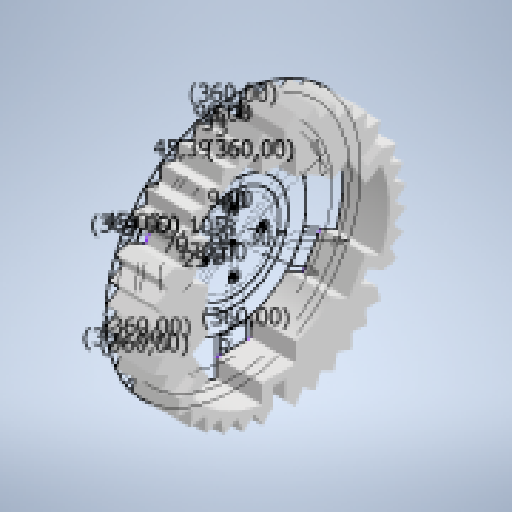
# Autodesk Inventor part: wheel
Saved by Autodesk Inventor 2023 (Build 270158000, 158)
## iProperties
Created: 2026-02-20
Part Number: wheel
Material: Типовые
Document SubType Name: Modeling
Designer: garin
Density: 1 g/cm^3
Appearance: По умолчанию
Author: garin
Autodesk Inventor part; units mm, degrees
ref_plane "YZ Plane" through (0, 0, 0) normal (1, 0, 0) x (0, 1, 0)
ref_plane "XZ Plane" through (0, 0, 0) normal (0, 1, 0) x (-1, 0, 0)
ref_plane "XY Plane" through (0, 0, 0) normal (0, 0, 1) x (1, 0, 0)
ref_plane "РабПлоскость1" through (-2, -29.6838, -23.3604) normal (-1, 0, 0) x (0, 0, 1)
sketch "Эскиз1" plane through (0, 0, 0) normal (1, 0, 0) x (0, 1, 0)
  circle A0 centre (0, 0) radius 35
  circle A1 centre (0, 0) radius 20
  line L0 (0, 0) -> (34.5691, 5.4752) construction
  line L1 (0, 0) -> (35, 0) construction
  line L2 (0, 0) -> (34.5691, -5.4752) construction
  line L3 (34.5691, 5.4752) -> (29.6307, 4.693) construction
  line L4 (29.6307, 4.693) -> (19.4416, 4.693)
  line L5 (19.4416, 4.693) -> (34.6839, 4.693)
  line L6 (19.4416, -4.693) -> (34.6839, -4.693)
  line L7 (13.7851, 14.4904) -> (21.4063, 27.6907) construction
  line L8 (10.751, 28.0074) -> (5.6565, 19.1834) construction
  line L9 (5.6565, 19.1834) -> (13.2777, 32.3837) construction
  line L10 (-5.6565, 19.1834) -> (-13.2777, 32.3837) construction
  line L11 (-18.8796, 23.3144) -> (-13.7851, 14.4904) construction
  line L12 (-13.7851, 14.4904) -> (-21.4063, 27.6907) construction
  line L13 (-19.4416, 4.693) -> (-34.6839, 4.693) construction
  line L14 (-29.6307, -4.693) -> (-19.4416, -4.693) construction
  line L15 (-19.4416, -4.693) -> (-34.6839, -4.693) construction
  line L16 (-13.7851, -14.4904) -> (-21.4063, -27.6907) construction
  line L17 (-10.751, -28.0074) -> (-5.6565, -19.1834) construction
  line L18 (-5.6565, -19.1834) -> (-13.2777, -32.3837) construction
  line L19 (5.6565, -19.1834) -> (13.2777, -32.3837) construction
  line L20 (18.8796, -23.3144) -> (13.7851, -14.4904) construction
  line L21 (13.7851, -14.4904) -> (21.4063, -27.6907) construction
  line L22 (0, 0) -> (17.5, 30.3109) construction
  line L23 (0, 0) -> (-17.5, 30.3109) construction
  line L24 (0, 0) -> (-35, 0) construction
  line L25 (0, 0) -> (-17.5, -30.3109) construction
  line L26 (0, 0) -> (17.5, -30.3109) construction
  line L27 (34.6839, 4.693) -> (29.6839, 4.693) construction
  line L28 (29.6839, 4.693) -> (29.6839, -4.693)
  line L29 (29.6839, 4.693) -> (29.6839, 1.693)
  line L30 (29.6839, 1.693) -> (34.959, 1.693)
  line L31 (29.6839, -4.693) -> (29.6839, -1.693) construction
  line L32 (29.6839, -1.693) -> (34.959, -1.693)
  line L33 (13.7851, 14.4904) -> (21.4063, 27.6907)
  line L34 (10.751, 28.0074) -> (5.6565, 19.1834)
  line L35 (13.3758, 26.5536) -> (16.0133, 31.1219)
  line L36 (5.6565, 19.1834) -> (13.2777, 32.3837)
  line L37 (10.7777, 28.0536) -> (18.9063, 23.3605)
  line L38 (16.3082, 24.8605) -> (18.9457, 29.4289)
  line L39 (-5.6565, 19.1834) -> (-13.2777, 32.3837)
  line L40 (-18.8796, 23.3144) -> (-13.7851, 14.4904)
  line L41 (-16.3082, 24.8605) -> (-18.9457, 29.4289)
  line L42 (-13.7851, 14.4904) -> (-21.4063, 27.6907)
  line L43 (-18.9063, 23.3605) -> (-10.7777, 28.0536)
  line L44 (-13.3758, 26.5536) -> (-16.0133, 31.1219)
  line L45 (-19.4416, 4.693) -> (-34.6839, 4.693)
  line L46 (-29.6307, -4.693) -> (-19.4416, -4.693)
  line L47 (-29.6839, -1.693) -> (-34.959, -1.693)
  line L48 (-19.4416, -4.693) -> (-34.6839, -4.693)
  line L49 (-29.6839, -4.693) -> (-29.6839, 4.693)
  line L50 (-29.6839, 1.693) -> (-34.959, 1.693)
  line L51 (-13.7851, -14.4904) -> (-21.4063, -27.6907)
  line L52 (-10.751, -28.0074) -> (-5.6565, -19.1834)
  line L53 (-13.3758, -26.5536) -> (-16.0133, -31.1219)
  line L54 (-5.6565, -19.1834) -> (-13.2777, -32.3837)
  line L55 (-10.7777, -28.0536) -> (-18.9063, -23.3605)
  line L56 (-16.3082, -24.8605) -> (-18.9457, -29.4289)
  line L57 (5.6565, -19.1834) -> (13.2777, -32.3837)
  line L58 (18.8796, -23.3144) -> (13.7851, -14.4904)
  line L59 (16.3082, -24.8605) -> (18.9457, -29.4289)
  line L60 (13.7851, -14.4904) -> (21.4063, -27.6907)
  line L61 (18.9063, -23.3605) -> (10.7777, -28.0536)
  line L62 (13.3758, -26.5536) -> (16.0133, -31.1219)
  circle A2 centre (0, 0) radius 30.0525
  line L63 (21.4063, 27.6907) -> (19.9063, 25.0926) construction
  line L64 (18.9457, 29.4289) -> (17.4457, 26.8308) construction
  line L65 (17.4457, 26.8308) -> (21.2118, 27.8399)
  line L66 (0, 0) -> (21.2118, 27.8399) construction
  line L67 (21.2384, 23.9411) -> (21.2118, 27.8399)
  line L68 (24.7499, 20.2901) -> (25.3388, 24.1443)
  line L69 (21.4607, 23.742) -> (25.3388, 24.1443)
  line L70 (27.6414, 16.1308) -> (28.831, 19.8437)
  line L71 (24.938, 20.0584) -> (28.831, 19.8437)
  line L72 (29.8403, 11.5673) -> (31.6009, 15.046)
  line L73 (27.7906, 15.8723) -> (31.6009, 15.046)
  line L74 (31.2917, 6.714) -> (33.5791, 9.8714)
  line L75 (29.9469, 11.2885) -> (33.5791, 9.8714)
  line L76 (31.9591, 1.6925) -> (34.716, 4.4494)
  line L77 (31.3529, 6.4219) -> (34.716, 4.4494)
  circle A3 centre (0, 0) radius 32.0038
  line L78 (-14.5133, 28.5238) -> (-13.5042, 32.2899)
  line L79 (-10.1144, 30.3635) -> (-13.5042, 32.2899)
  line L80 (-9.8308, 30.4565) -> (-8.2401, 34.0162)
  line L81 (-5.1968, 31.5791) -> (-8.2401, 34.0162)
  line L82 (14.5138, 28.5236) -> (13.5047, 32.2897)
  line L83 (10.1149, 30.3634) -> (13.5047, 32.2897)
  line L84 (9.8313, 30.4564) -> (8.2407, 34.016)
  line L85 (5.1973, 31.579) -> (8.2407, 34.016)
  line L86 (4.9026, 31.6261) -> (2.7702, 34.8902)
  line L87 (0.1495, 32.0035) -> (2.7702, 34.8902)
  line L88 (-0.149, 32.0035) -> (-2.7697, 34.8902)
  line L89 (-4.9021, 31.6262) -> (-2.7697, 34.8902)
  line L90 (-31.959, 1.693) -> (-34.716, 4.45)
  line L91 (-31.3528, 6.4224) -> (-34.716, 4.45)
  line L92 (-31.2916, 6.7145) -> (-33.5789, 9.8719)
  line L93 (-29.9467, 11.289) -> (-33.5789, 9.8719)
  line L94 (-17.4453, 26.8311) -> (-21.2113, 27.8403)
  line L95 (-21.238, 23.9415) -> (-21.2113, 27.8403)
  line L96 (-21.4603, 23.7424) -> (-25.3384, 24.1447)
  line L97 (-24.7496, 20.2905) -> (-25.3384, 24.1447)
  line L98 (-24.9377, 20.0588) -> (-28.8307, 19.8442)
  line L99 (-27.6411, 16.1312) -> (-28.8307, 19.8442)
  line L100 (-27.7903, 15.8727) -> (-31.6007, 15.0465)
  line L101 (-29.8401, 11.5678) -> (-31.6007, 15.0465)
  line L102 (-17.4457, -26.8308) -> (-21.2118, -27.8399)
  line L103 (-21.2384, -23.9411) -> (-21.2118, -27.8399)
  line L104 (-21.4607, -23.742) -> (-25.3388, -24.1443)
  line L105 (-24.7499, -20.2901) -> (-25.3388, -24.1443)
  line L106 (-31.9591, -1.6925) -> (-34.716, -4.4494)
  line L107 (-31.3529, -6.4219) -> (-34.716, -4.4494)
  line L108 (-31.2917, -6.714) -> (-33.5791, -9.8714)
  line L109 (-29.9469, -11.2885) -> (-33.5791, -9.8714)
  line L110 (-29.8403, -11.5673) -> (-31.6009, -15.046)
  line L111 (-27.7906, -15.8723) -> (-31.6009, -15.046)
  line L112 (-27.6414, -16.1308) -> (-28.831, -19.8437)
  line L113 (-24.938, -20.0584) -> (-28.831, -19.8437)
  line L114 (14.5133, -28.5238) -> (13.5042, -32.2899)
  line L115 (10.1144, -30.3635) -> (13.5042, -32.2899)
  line L116 (9.8308, -30.4565) -> (8.2401, -34.0162)
  line L117 (5.1968, -31.5791) -> (8.2401, -34.0162)
  line L118 (-14.5138, -28.5236) -> (-13.5047, -32.2897)
  line L119 (-10.1149, -30.3634) -> (-13.5047, -32.2897)
  line L120 (-9.8313, -30.4564) -> (-8.2407, -34.016)
  line L121 (-5.1973, -31.579) -> (-8.2407, -34.016)
  line L122 (-4.9026, -31.6261) -> (-2.7702, -34.8902)
  line L123 (-0.1495, -32.0035) -> (-2.7702, -34.8902)
  line L124 (0.149, -32.0035) -> (2.7697, -34.8902)
  line L125 (4.9021, -31.6262) -> (2.7697, -34.8902)
  line L126 (31.959, -1.693) -> (34.716, -4.45)
  line L127 (31.3528, -6.4224) -> (34.716, -4.45)
  line L128 (31.2916, -6.7145) -> (33.5789, -9.8719)
  line L129 (29.9467, -11.289) -> (33.5789, -9.8719)
  line L130 (17.4453, -26.8311) -> (21.2113, -27.8403)
  line L131 (21.238, -23.9415) -> (21.2113, -27.8403)
  line L132 (21.4603, -23.7424) -> (25.3384, -24.1447)
  line L133 (24.7496, -20.2905) -> (25.3384, -24.1447)
  line L134 (24.9377, -20.0588) -> (28.8307, -19.8442)
  line L135 (27.6411, -16.1312) -> (28.8307, -19.8442)
  line L136 (27.7903, -15.8727) -> (31.6007, -15.0465)
  line L137 (29.8401, -11.5678) -> (31.6007, -15.0465)
  circle A4 centre (0, 0) radius 11 construction
  line L138 (0, 0) -> (0, 8) construction
  circle A5 centre (0, 8) radius 1.5
  circle A6 centre (0, -8) radius 1.5
  line L139 (0, 0) -> (8, 0) construction
  circle A7 centre (8, 0) radius 1.5
  circle A8 centre (-8, 0) radius 1.5
  circle A9 centre (0, 0) radius 12.5
  circle A10 centre (0, 0) radius 15
  line L140 (0, 0) -> (-19.6962, 3.473) construction
  line L141 (0, 0) -> (20, 0) construction
  line L142 (-19.6962, 3.473) -> (-19.6962, -3.473)
  line L143 (-19.6962, -3.473) -> (0, 0) construction
  line L144 (-19.6962, 3.473) -> (-24.6962, 3.473)
  line L145 (-24.6962, 3.473) -> (-24.6962, -3.473)
  line L146 (-24.6962, -3.473) -> (-19.6962, -3.473)
  line L147 (-12.8558, 15.3209) -> (0, 0) construction
  line L148 (0, 0) -> (-6.8404, 18.7939) construction
  line L149 (-6.8404, 18.7939) -> (-9.3404, 23.124)
  line L150 (-9.3404, 23.124) -> (-15.3558, 19.651)
  line L151 (-15.3558, 19.651) -> (-12.8558, 15.3209)
  line L152 (6.8404, 18.7939) -> (0, 0) construction
  line L153 (0, 0) -> (12.8558, 15.3209) construction
  line L154 (12.8558, 15.3209) -> (15.3558, 19.651)
  line L155 (15.3558, 19.651) -> (9.3404, 23.124)
  line L156 (9.3404, 23.124) -> (6.8404, 18.7939)
  line L157 (19.6962, 3.473) -> (0, 0) construction
  line L158 (0, 0) -> (19.6962, -3.473) construction
  line L159 (19.6962, -3.473) -> (24.6962, -3.473)
  line L160 (24.6962, -3.473) -> (24.6962, 3.473)
  line L161 (24.6962, 3.473) -> (19.6962, 3.473)
  line L162 (12.8558, -15.3209) -> (0, 0) construction
  line L163 (0, 0) -> (6.8404, -18.7939) construction
  line L164 (6.8404, -18.7939) -> (9.3404, -23.124)
  line L165 (9.3404, -23.124) -> (15.3558, -19.651)
  line L166 (15.3558, -19.651) -> (12.8558, -15.3209)
  line L167 (-6.8404, -18.7939) -> (0, 0) construction
  line L168 (0, 0) -> (-12.8558, -15.3209) construction
  line L169 (-12.8558, -15.3209) -> (-15.3558, -19.651)
  line L170 (-15.3558, -19.651) -> (-9.3404, -23.124)
  line L171 (-9.3404, -23.124) -> (-6.8404, -18.7939)
  line L172 (-13.3758, 26.5536) -> (-10.8819, 22.234)
  line L173 (-16.4686, 25.1384) -> (-13.8143, 20.541)
  line L174 (-30.0048, -1.693) -> (-24.6962, -1.693)
  line L175 (-29.6839, 1.693) -> (-24.6962, 1.693)
  line L176 (-13.5362, -26.8314) -> (-10.8819, -22.234)
  line L177 (-16.3082, -24.8605) -> (-13.8143, -20.541)
  line L178 (16.4686, -25.1384) -> (13.8143, -20.541)
  line L179 (13.3758, -26.5536) -> (10.8819, -22.234)
  line L180 (30.0048, 1.693) -> (24.6962, 1.693)
  line L181 (29.6839, -1.693) -> (24.6962, -1.693)
  line L182 (13.5362, 26.8314) -> (10.8819, 22.234)
  line L183 (16.3082, 24.8605) -> (13.8143, 20.541)
  circle A11 centre (0, 0) radius 20
  line L184 (-10.8819, 22.234) -> (-12.0277, 24.2186)
  line L185 (-12.0277, 24.2186) -> (-14.9601, 22.5256)
  line L186 (-26.9878, 1.693) -> (-26.9878, -1.693)
  line L187 (-14.9601, -22.5256) -> (-12.0277, -24.2186)
  line L188 (12.0277, -24.2186) -> (14.9601, -22.5256)
  line L189 (26.9878, -1.693) -> (26.9878, 1.693)
  line L190 (14.9601, 22.5256) -> (12.0277, 24.2186)
  line L191 (-8.2838, 23.734) -> (-16.4124, 19.041)
  line L192 (-24.6962, 4.693) -> (-24.6962, -4.693)
  line L193 (-16.4124, -19.041) -> (-8.2838, -23.734)
  line L194 (8.2838, -23.734) -> (16.4124, -19.041)
  line L195 (24.6962, -4.693) -> (24.6962, 4.693)
  line L196 (16.4124, 19.041) -> (8.2838, 23.734)
  point P0 (-14.5133, -28.5238)
  point P1 (-14.5136, -28.5243)
  point P2 (14.5133, -28.5238)
  point P3 (17.4457, -26.8308)
  point P4 (17.446, -26.8313)
  point P5 (31.959, -1.693)
  point P6 (31.959, 1.693)
  point P7 (31.9596, 1.693)
  point P8 (14.5133, 28.5238)
  point P9 (14.5136, 28.5243)
  point P10 (-14.5133, 28.5238)
  point P11 (-17.4457, 26.8308)
  point P12 (-17.446, 26.8313)
  point P13 (-31.959, 1.693)
  point P14 (-31.959, -1.693)
  point P15 (-31.9596, -1.693)
  point P16 (-17.4457, -26.8308)
  point P17 (-18.9055, -23.3609)
  point P18 (-10.7784, -28.0531)
  point P19 (18.9055, -23.3609)
  point P20 (10.7784, -28.0531)
  point P21 (29.6839, 4.6922)
  point P22 (29.6839, -4.6922)
  point P23 (10.7784, 28.0531)
  point P24 (18.9055, 23.3609)
  point P25 (-10.7784, 28.0531)
  point P26 (-18.9055, 23.3609)
  point P27 (-29.6839, -4.6922)
  point P28 (-29.6839, 4.6922)
  point P29 (18.9062, 23.3604)
  point P30 (-18.9062, 23.3604)
  point P31 (-29.6838, 4.693)
  point P32 (-10.7776, -28.0534)
  point P33 (10.7776, -28.0534)
  point P34 (29.6838, 4.693)
  point P35 (-14.5133, 28.5238)
  point P36 (-31.959, 1.693)
  point P37 (-17.4457, -26.8308)
  point P38 (14.5133, -28.5238)
  point P39 (31.959, -1.693)
  dimension "d129" = 60.105
  dimension "d109" = 70
  dimension "d110" = 40
  dimension "d111" = 9
  dimension "d112" = 5
  dimension "d115" = 360
  dimension "d119" = 360
  dimension "d121" = 5
  dimension "d122" = 90
  dimension "d123" = 3
  dimension "d124" = 3
  dimension "d127" = 360
  dimension "d132" = 3
  dimension "d133" = 45
  dimension "d136" = 45.392
  dimension "d140" = 360
  dimension "d168" = 22
  dimension "d169" = 8
  dimension "d170" = 3
  dimension "d171" = 8
  dimension "d172" = 3
  dimension "d173" = 25
  dimension "d176" = 30
  dimension "d179" = 170
  dimension "d180" = 5
  dimension "d183" = 360
  dimension "d187" = 360
  dimension "d191" = 360
  dimension "d195" = 360
  constraints: 394 end point, 50 point on line, 10 centre point, 9 coincident, 8 point on circle, 6 perpendicular, 6 symmetric about line, 4 horizontal, 2 equal length, 2 vertical, 522 other
  measures "d109" diameter of A0
  measures "d110" diameter of A1
  measures "d111" angle of L1 L0
  measures "d112" distance of L0.end L3.end
  measures "d121" distance of L5.end L27.end
  measures "d122" angle of L28 L27
  measures "d123" distance of L27.end L29.end
  measures "d124" distance of L28.end L31.end
  measures "d132" distance of L38.end L64.end
  measures "d133" angle of L65 L64
  measures "d168" diameter of A4
  measures "d169" distance of L138.start L138.end
  measures "d170" diameter of A5
  measures "d171" distance of L138.start L139.end
  measures "d172" diameter of A7
  measures "d173" diameter of A9
  measures "d176" diameter of A10
  measures "d179" angle of L141 L140
  measures "d180" distance of L140.end L144.end
ref_plane "РабПлоскость2" through (0, -34.716, -34.8902) normal (1, 0, 0) x (0, 1, 0)
extrude "Выдавливание1" add sketch "Эскиз1" along normal blind 12.5 from surface at 0 contours L76 A3 L5 L77 | L30 A2 L5 A3 | L127 L6 A3 L126 | A3 L6 A2 L32 | L5 A3 L77 | L30 L28 A2 | L5 A2 L33 A3 | L127 A3 L6 | A2 L28 L32 | A3 L60 A2 L6 | L74 A3 L75 | L129 A3 L128 | L72 A3 L73 | A2 L38 A3 L33 | L37 L38 A2 | L136 A3 L137 | A2 L59 L61 | L60 A3 L59 A2 | L70 A3 L71 | A3 L65 L67 L33 | L33 L67 A3 | L134 A3 L135 | A3 L131 L60 | L60 L131 L130 A3 | L68 A3 L69 | L37 A2 L35 | A2 L36 A3 L35 | L132 A3 L133 | L62 A2 L61 | L62 A3 L57 A2 | A3 L36 L83 L82 | A2 L39 A3 L36 | L114 L115 L57 A3 | L57 A3 L54 A2 | A3 L83 L36 | A2 L44 A3 L39 | L43 L44 A2 | L57 L115 A3 | A2 L53 L55 | L54 A3 L53 A2 | A3 L78 L79 L39 | L39 L79 A3 | A3 L119 L54 | L54 L119 L118 A3 | A3 L85 L84 | L43 A2 L41 | A2 L42 A3 L41 | L116 L117 A3 | L56 A2 L55 | L56 A3 L51 A2 | L86 A3 L87 | L80 L81 A3 | A3 L42 L95 L94 | A2 L45 A3 L42 | L124 A3 L125 | L102 L103 L51 A3 | A3 L121 L120 | L51 A3 L48 A2 | L88 A3 L89 | A3 L95 L42 | A2 L50 A3 L45 | L49 L50 A2 | L122 A3 L123 | L51 L103 A3 | A2 L47 L49 | L48 A3 L47 A2 | A3 L90 L91 L45 | L45 L91 A3 | A3 L107 L48 | L48 L107 L106 A3 | A3 L97 L96 | L104 L105 A3 | L98 A3 L99 | L92 L93 A3 | L112 A3 L113 | A3 L109 L108 | L100 A3 L101 | L110 A3 L111
extrude "Выдавливание2" add sketch "Эскиз1" along normal blind 12.5 contours L180 L160 L195 L4 L5 L28 | L28 L6 L195 L160 L181 | A2 L60 L58 A1 L6 | L189 L181 L160 L180 | L33 L196 L155 L183 L37 | L61 L178 L165 L194 L58 L60 | L182 L155 L196 L34 L36 L37 | L183 L155 L182 L190 | L61 L57 L194 L165 L179 | L188 L179 L165 L178 | L36 L34 A1 L39 A2 | L39 L191 L150 L172 L43 | L55 L176 L170 L193 L52 L54 | L173 L150 L191 L40 L42 L43 | L172 L150 L173 L185 | L55 L51 L193 L170 L177 | L187 L177 L170 L176 | A2 L48 L46 A1 L51 | L45 L192 L145 L175 L49 | L49 L174 L145 L192 L46 L48 | L175 L145 L174 L186
